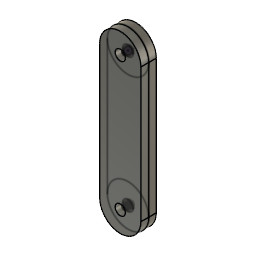
FiveBarLinkage (Autodesk Fusion 360 archive; units mm, degrees)
design "PassiveLink"
part number: 2026-02-01-17-53-22-850
Autodesk Fusion 360 part; units mm, degrees
sketch "Sketch1" plane through (0, 0, 0) normal (0, 1, 0) x (1, 0, 0)
  circle A0 centre (0, 0) radius 20
  line L0 (-20, 0) -> (-20, 130)
  line L1 (20, 130) -> (20, 0)
  circle A1 centre (0, 130) radius 20
  circle A2 centre (0, 0) radius 5
  circle A3 centre (0, 130) radius 5
  dimension "d1" = 40
  dimension "d3" = 40
  dimension "d5" = 20
  dimension "d6" = 130
  dimension "d9" = 10
  dimension "d10" = 10
  constraint coincident A0.centre A2.centre
  constraint coincident A0 L0.start
  constraint tangent A0 L0
  constraint vertical L0
  constraint coincident A0 L1.end
  constraint tangent A0 L1
  constraint coincident A1 L1.start
  constraint coincident A1 L0.end
  constraint tangent L1 A1
  constraint concentric A0 A2
  constraint concentric A1 A3
  measures "d1" diameter of A0
  measures "d3" diameter of A1
  measures "d5" distance of L0 A1.centre
  measures "d6" distance of L1.end L1.start
  measures "d9" diameter of A2
  measures "d10" diameter of A3
extrude "Extrude1" add sketch "Sketch1" along normal mid plane 15 contours A0 | A0 L0 L1 A1 | A1 | A2 | A3
extrude "Extrude2" cut sketch "Sketch1" along normal through all and the other way through all contours A2 | A3

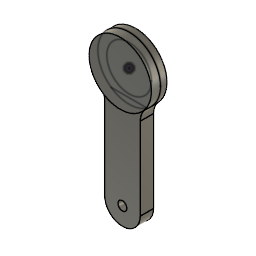
design "InputLink2"
part number: 2026-02-01-16-20-52-191
Autodesk Fusion 360 part; units mm, degrees
sketch "Sketch1" plane through (0, 0, 0) normal (0, 1, 0) x (1, 0, 0)
  circle A0 centre (0, 0) radius 35
  circle A1 centre (0, 0) radius 25
  line L0 (-20, 28.7228) -> (20, 28.7228)
  dimension "d1" = 70
  dimension "d2" = 50
  dimension "d3" = 40
  constraint coincident A0.centre A1.centre
  constraint concentric A0 A1
  constraint coincident A0 L0.start
  constraint coincident A0 L0.end
  constraint horizontal L0
  measures "d1" diameter of A0
  measures "d2" diameter of A1
  measures "d3" distance of L0.start L0.end
extrude "Extrude1" add sketch "Sketch1" along normal blind 7.5 and the other way blind 10
ref_plane "WorkPlane1" through (0, 0, -50) normal (0, 0, 1) x (1, 0, 0)
sketch "Sketch2" plane through (0, 0, -50) normal (0, 0, 1) x (1, 0, 0)
  line L0 (20, 7.5) -> (-20, 7.5)
  line L1 (-20, 7.5) -> (-20, -7.5)
  line L2 (-20, -7.5) -> (20, -7.5)
  line L3 (20, -7.5) -> (20, 7.5)
  line L4 (20, 7.5) -> (-20, -7.5) construction
  line L5 (-20, 7.5) -> (20, -7.5) construction
  dimension "d7" = 40
  dimension "d8" = 15
  constraint horizontal L0
  constraint perpendicular L0 L1
  constraint parallel L0 L2
  constraint parallel L1 L3
  constraint coincident L4 origin
  constraint coincident L5 origin
  measures "d7" distance of L1.end L2.end
  measures "d8" distance of L0.end L1.end
extrude "Extrude2" add sketch "Sketch2" along normal blind 23 and the other way blind 100
fillet "Fillet1" radius 20 2 edges at (20, 0, -28.7228) (-20, 0, -28.7228)
fillet "Fillet1" radius 20 2 edges at (20, 0, -150) (-20, 0, -150)
sketch "Sketch3" plane through (0, -7.5, 0) normal (0, -1, 0) x (1, 0, 0)
  arc A0 (-20, -130) -> (20, -130) centre (0, -130) ccw
  line L0 (20, -130) -> (20, -37.7492)
  arc A1 (25.4545, -24.0222) -> (20, -37.7492) centre (40, -37.7492) ccw
  arc A2 (-25.4545, -24.0222) -> (25.4545, -24.0222) centre (0, 0) ccw
  arc A3 (-20, -37.7492) -> (-25.4545, -24.0222) centre (-40, -37.7492) ccw
  line L1 (-20, -37.7492) -> (-20, -130)
  circle A4 centre (0, -130) radius 5
  dimension "d17" = 10
  constraint concentric A0 A4
  measures "d17" diameter of A4
extrude "Extrude3" cut sketch "Sketch3" against normal through all contours A4
extrude "Extrude5" add sketch "Sketch1" against normal blind 10 contours A1
extrude "Extrude6" cut sketch "Sketch1" against normal blind 2.5 contours A1

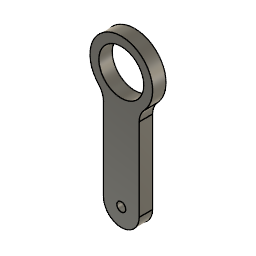
design "InputLink1"
part number: 2026-02-01-16-20-52-191
Autodesk Fusion 360 part; units mm, degrees
sketch "Sketch1" plane through (0, 0, 0) normal (0, 1, 0) x (1, 0, 0)
  circle A0 centre (0, 0) radius 35
  circle A1 centre (0, 0) radius 25
  line L0 (-20, 28.7228) -> (20, 28.7228)
  dimension "d1" = 70
  dimension "d2" = 50
  dimension "d3" = 40
  constraint coincident A0.centre A1.centre
  constraint concentric A0 A1
  constraint coincident A0 L0.start
  constraint coincident A0 L0.end
  constraint horizontal L0
  measures "d1" diameter of A0
  measures "d2" diameter of A1
  measures "d3" distance of L0.start L0.end
extrude "Extrude1" add sketch "Sketch1" along normal mid plane 15
ref_plane "WorkPlane1" through (0, 0, -50) normal (0, 0, 1) x (1, 0, 0)
sketch "Sketch2" plane through (0, 0, -50) normal (0, 0, 1) x (1, 0, 0)
  line L0 (20, 7.5) -> (-20, 7.5)
  line L1 (-20, 7.5) -> (-20, -7.5)
  line L2 (-20, -7.5) -> (20, -7.5)
  line L3 (20, -7.5) -> (20, 7.5)
  line L4 (20, 7.5) -> (-20, -7.5) construction
  line L5 (-20, 7.5) -> (20, -7.5) construction
  dimension "d7" = 40
  dimension "d8" = 15
  constraint horizontal L0
  constraint perpendicular L0 L1
  constraint parallel L0 L2
  constraint parallel L1 L3
  constraint coincident L4 origin
  constraint coincident L5 origin
  measures "d7" distance of L1.end L2.end
  measures "d8" distance of L0.end L1.end
extrude "Extrude2" add sketch "Sketch2" along normal blind 23 and the other way blind 100
fillet "Fillet1" radius 20 2 edges at (20, 0, -28.7228) (-20, 0, -28.7228)
fillet "Fillet1" radius 20 2 edges at (20, 0, -150) (-20, 0, -150)
sketch "Sketch3" plane through (0, -7.5, 0) normal (0, -1, 0) x (1, 0, 0)
  circle A0 centre (0, 0) radius 25
  arc A1 (-20, -130) -> (20, -130) centre (0, -130) ccw
  line L0 (20, -130) -> (20, -37.7492)
  arc A2 (25.4545, -24.0222) -> (20, -37.7492) centre (40, -37.7492) ccw
  arc A3 (25.4545, -24.0222) -> (-25.4545, -24.0222) centre (0, 0) ccw
  arc A4 (-20, -37.7492) -> (-25.4545, -24.0222) centre (-40, -37.7492) ccw
  line L1 (-20, -37.7492) -> (-20, -130)
  circle A5 centre (0, -130) radius 5
  dimension "d17" = 10
  constraint concentric A1 A5
  measures "d17" diameter of A5
extrude "Extrude3" cut sketch "Sketch3" against normal through all contours A5
